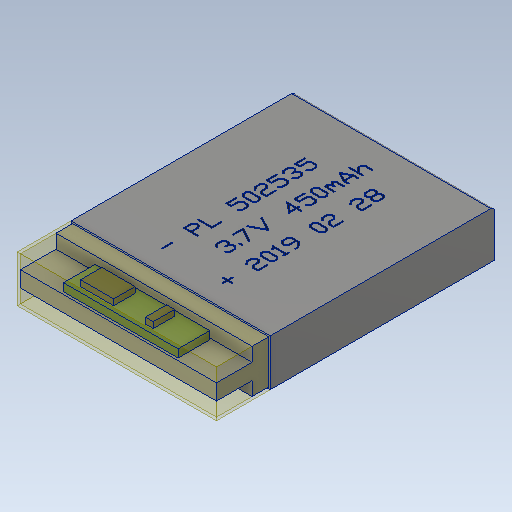
# Autodesk Inventor part: LiPo 502535
Saved by Autodesk Inventor 2020.1 (Build 241239000, 239)
## iProperties
Created: 2019-07-15
Part Number: LiPo 502535
Material: Generic
Document SubType Name: Modeling
Designer: Petar
Density: 1 g/cm^3
Appearance: Default
Mass: 4.91007 g
Surface Area: 36.002 cm^2
Volume: 4.91007 cm^3
Author: Petar
Autodesk Inventor part; units mm, degrees
ref_plane "YZ Plane" through (0, 0, 0) normal (1, 0, 0) x (0, 1, 0)
ref_plane "XZ Plane" through (0, 0, 0) normal (0, 1, 0) x (-1, 0, 0)
sketch "Sketch1" plane through (0, 0, 0) normal (0, 1, 0) x (-1, 0, 0)
  line L0 (-12.6, -17.5205) -> (12.6, -17.5205)
  line L1 (12.6, -17.5205) -> (12.6, 12.9793)
  line L2 (12.5, 17.4793) -> (-12.5, 17.4793)
  line L3 (-12.5, 17.4793) -> (-12.5, 12.9793)
  line L4 (12.5, 12.9793) -> (-12.5, 12.9793)
  line L5 (12.5, 12.9793) -> (12.5, 17.4793)
  line L6 (-12.6, 12.9793) -> (-12.6, -17.5205)
  line L7 (0, -17.5205) -> (0, 12.9793) construction
  line L8 (12.6, 12.9793) -> (12.5, 12.9793)
  line L9 (-12.6, 12.9793) -> (-12.5, 12.9793)
  point P0 (0, 0)
  dimension "d1" = 35
  dimension "d2" = 4.5
  dimension "d12" = 25.2
  dimension "d13" = 25
  constraints: 20 end point, 5 parallel, 4 perpendicular, 2 horizontal, 2 midpoint, 1 collinear, 1 vertical
  measures "d1" distance of L2.start L0.end
  measures "d2" distance between parallel lines of L2 L4
  measures "d12" distance between parallel lines of L6 L1
  measures "d13" distance between parallel lines of L5 L3
extrude "Extrusion1" add sketch "Sketch1" along normal mid plane 5.9 contours L6 L9 L4 L8 L1 L0
extrude "Extrusion2" add sketch "Sketch1" along normal mid plane 2 contours L3 L2 L5 L4
ref_plane "Work Plane1" through (-12.5, 1, 17.6793) normal (0, 0, 1) x (1, 0, 0)
sketch "Sketch3" plane through (-12.5, 1, 17.6793) normal (0, 0, 1) x (1, 0, 0)
  line L0 (25, -2) -> (0, -2) construction
  line L1 (0, -2) -> (0, 0) construction
  line L2 (0, 0) -> (25, 0) construction
  line L3 (25, 0) -> (25, -2) construction
  line L4 (25.1, -3.95) -> (25.1, 1.95) projected
  line L5 (-0.1, 1.95) -> (25.1, 1.95) projected
  line L6 (-0.1, -3.95) -> (-0.1, 1.95) projected
  line L7 (25.1, -3.95) -> (-0.1, -3.95) projected
  line L8 (24.9, 1.75) -> (24.9, -3.75)
  line L9 (24.9, -3.75) -> (0.1, -3.75)
  line L10 (0.1, -3.75) -> (0.1, 1.75)
  line L11 (0.1, 1.75) -> (24.9, 1.75)
  point P0 (12.5, -1)
  dimension "d17" = 0.2
  constraints: 8 end point, 3 other
  measures "d17" distance between parallel lines of L5 L11
extrude "Extrusion4" cut sketch "Sketch3" against normal blind 6.8
extrude "Extrusion5" add sketch "Sketch3" against normal up to next separate body
extrude "Extrusion6" add sketch "Sketch3" against normal blind 0.2 contours L8 L9 L10 L11 bodies 2
sketch "Sketch4" plane through (0, 1, 0) normal (0, 1, 0) x (1, 0, 0)
  line L0 (-7.25, -17.1793) -> (7.25, -17.1793)
  line L1 (7.25, -17.1793) -> (7.25, -13.1793)
  line L2 (7.25, -13.1793) -> (-7.25, -13.1793)
  line L3 (-7.25, -13.1793) -> (-7.25, -17.1793)
  line L4 (0, -17.1793) -> (0, -13.1793) construction
  line L5 (12.4, -17.4793) -> (12.4, -12.9793) construction
  line L6 (-12.4, -12.9793) -> (-12.4, -17.4793) construction
  line L7 (-12.4, -12.9793) -> (12.4, -12.9793) construction
  point P0 (0, 0)
  dimension "d24" = 14.5
  dimension "d25" = 4
  dimension "d26" = 24.8
  dimension "d27" = 12.4
  dimension "d28" = 0.2
  constraints: 10 end point, 2 midpoint, 2 parallel, 1 horizontal, 1 perpendicular
  measures "d24" distance of L2.end L1.end
  measures "d25" distance of L1.end L0.end
  measures "d26" distance between parallel lines of L5 L6
  measures "d27" distance between parallel lines of L5 L4
  measures "d28" distance between parallel lines of L7 L2
extrude "Extrusion7" add sketch "Sketch4" along normal blind 1 bodies 1
sketch "Sketch5" plane through (0, 2, 0) normal (0, 1, 0) x (1, 0, 0)
  line L0 (2.45, -16.5293) -> (3.45, -16.5293)
  line L1 (3.45, -16.5293) -> (3.45, -13.8293)
  line L2 (3.45, -13.8293) -> (2.45, -13.8293)
  line L3 (2.45, -13.8293) -> (2.45, -16.5293)
  line L4 (-5.75, -16.5293) -> (-1.55, -16.5293)
  line L5 (-1.55, -16.5293) -> (-1.55, -13.8293)
  line L6 (-1.55, -13.8293) -> (-5.75, -13.8293)
  line L7 (-5.75, -13.8293) -> (-5.75, -16.5293)
  line L8 (-5.75, -15.1793) -> (-1.55, -15.1793) construction
  line L9 (2.45, -15.1793) -> (3.45, -15.1793) construction
  line L10 (-7.25, -17.1793) -> (7.25, -17.1793) construction
  line L11 (7.25, -17.1793) -> (7.25, -13.1793) construction
  line L12 (-7.25, -13.1793) -> (-7.25, -17.1793) construction
  point P0 (0, 0)
  dimension "d31" = 1
  dimension "d33" = 4.2
  dimension "d34" = 2.7
  dimension "d35" = 2
  dimension "d36" = 3.8
  dimension "d37" = 1.5
  constraints: 20 end point, 5 parallel, 4 midpoint, 2 horizontal, 2 perpendicular, 1 collinear
  measures "d31" distance of L2.end L1.end
  measures "d33" distance of L6.end L5.end
  measures "d34" distance of L5.end L4.end
  measures "d35" distance between parallel lines of L10 L8
  measures "d36" distance between parallel lines of L11 L1
  measures "d37" distance between parallel lines of L12 L7
extrude "Extrusion8" add sketch "Sketch5" along normal up to surface (0.75 mm away) bodies 1
sketch "Sketch6" plane through (0, 2.95, 0) normal (0, 1, 0) x (1, 0, 0)
  line L0 (-12.6, -8.3793) -> (-12.6, 17.5205) construction
  line L1 (-12.6, 17.5205) -> (12.6, 17.5205) construction
  line L2 (12.6, 17.5205) -> (12.6, -8.3793) construction
  line L3 (12.6, -8.3793) -> (-12.6, -8.3793) construction
  line L4 (12.6, 17.5205) -> (-12.6, 17.5205) construction
  line L5 (-12.6, 17.5205) -> (-12.6, -10.8793) construction
  line L6 (12.6, -10.8793) -> (12.6, 17.5205) construction
  line L7 (-12.6, -10.8793) -> (12.6, -10.8793) construction
  line L8 (-3.7334, -6.824) -> (-3.7334, -8.1408)
  line L9 (-3.7334, -8.1408) -> (-3.8859, -8.1408)
  line L10 (-3.8859, -8.1408) -> (-3.8859, -6.824)
  line L11 (-3.8859, -6.824) -> (-3.7334, -6.824)
  line L12 (-4.061, -3.2149) -> (-3.7334, -3.5622)
  line L13 (-3.7334, -3.5622) -> (-3.7334, -4.4109)
  line L14 (-3.7334, -4.4109) -> (-2.9104, -4.4109)
  line L15 (-2.9104, -4.4109) -> (-2.9104, -4.5725)
  line L16 (-2.9104, -4.5725) -> (-4.7285, -4.5725)
  line L17 (-4.7285, -4.5725) -> (-4.7285, -3.5622)
  line L18 (-4.7285, -3.5622) -> (-4.4038, -3.2149)
  line L19 (-4.4038, -3.2149) -> (-4.061, -3.2149)
  line L20 (-4.123, -3.378) -> (-4.3404, -3.378)
  line L21 (-4.3404, -3.378) -> (-4.5775, -3.6287)
  line L22 (-4.5775, -3.6287) -> (-4.5775, -4.4109)
  line L23 (-4.5775, -4.4109) -> (-3.8859, -4.4109)
  line L24 (-3.8859, -4.4109) -> (-3.8859, -3.6287)
  line L25 (-3.8859, -3.6287) -> (-4.123, -3.378)
  line L26 (-2.8938, -1.4421) -> (-2.8938, -2.7785)
  line L27 (-2.8938, -2.7785) -> (-4.7104, -2.7785)
  line L28 (-4.7104, -2.7785) -> (-4.7104, -2.6169)
  line L29 (-4.7104, -2.6169) -> (-3.0433, -2.6169)
  line L30 (-3.0433, -2.6169) -> (-3.0433, -1.4421)
  line L31 (-3.0433, -1.4421) -> (-2.8938, -1.4421)
  line L32 (-3.2169, 2.167) -> (-2.8938, 1.8196)
  line L33 (-2.8938, 1.8196) -> (-2.8938, 1.1552)
  line L34 (-2.8938, 1.1552) -> (-3.235, 0.7883)
  line L35 (-3.235, 0.7883) -> (-3.3438, 0.9045)
  line L36 (-3.3438, 0.9045) -> (-3.0433, 1.2217)
  line L37 (-3.0433, 1.2217) -> (-3.0433, 1.7532)
  line L38 (-3.0433, 1.7532) -> (-3.2788, 2.0039)
  line L39 (-3.2788, 2.0039) -> (-3.7802, 2.0039)
  line L40 (-3.7802, 2.0039) -> (-4.0157, 1.7532)
  line L41 (-4.0157, 1.7532) -> (-4.0157, 0.8094)
  line L42 (-4.0157, 0.8094) -> (-4.7285, 0.8094)
  line L43 (-4.7285, 0.8094) -> (-4.7285, 2.1458)
  line L44 (-4.7285, 2.1458) -> (-4.5775, 2.1458)
  line L45 (-4.5775, 2.1458) -> (-4.5775, 0.971)
  line L46 (-4.5775, 0.971) -> (-4.1683, 0.971)
  line L47 (-4.1683, 0.971) -> (-4.1683, 1.8196)
  line L48 (-4.1683, 1.8196) -> (-3.8421, 2.167)
  line L49 (-3.8421, 2.167) -> (-3.2169, 2.167)
  line L50 (-3.2169, 3.6604) -> (-2.8938, 3.3146)
  line L51 (-2.8938, 3.3146) -> (-2.8938, 2.9492)
  line L52 (-2.8938, 2.9492) -> (-3.2169, 2.6034)
  line L53 (-3.2169, 2.6034) -> (-4.4038, 2.6034)
  line L54 (-4.4038, 2.6034) -> (-4.7285, 2.9492)
  line L55 (-4.7285, 2.9492) -> (-4.7285, 3.3146)
  line L56 (-4.7285, 3.3146) -> (-4.4038, 3.6604)
  line L57 (-4.4038, 3.6604) -> (-3.2169, 3.6604)
  line L58 (-3.2788, 3.4988) -> (-4.3404, 3.4988)
  line L59 (-4.3404, 3.4988) -> (-4.5775, 3.2482)
  line L60 (-4.5775, 3.2482) -> (-4.5775, 3.0156)
  line L61 (-4.5775, 3.0156) -> (-4.3404, 2.765)
  line L62 (-4.3404, 2.765) -> (-3.2788, 2.765)
  line L63 (-3.2788, 2.765) -> (-3.0433, 3.0156)
  line L64 (-3.0433, 3.0156) -> (-3.0433, 3.2482)
  line L65 (-3.0433, 3.2482) -> (-3.2788, 3.4988)
  line L66 (-4.061, 5.4559) -> (-3.7334, 5.1086)
  line L67 (-3.7334, 5.1086) -> (-3.7334, 4.5106)
  line L68 (-3.7334, 4.5106) -> (-3.4978, 4.2599)
  line L69 (-3.4978, 4.2599) -> (-3.0433, 4.2599)
  line L70 (-3.0433, 4.2599) -> (-3.0433, 5.4347)
  line L71 (-3.0433, 5.4347) -> (-2.8938, 5.4347)
  line L72 (-2.8938, 5.4347) -> (-2.8938, 4.0983)
  line L73 (-2.8938, 4.0983) -> (-3.5597, 4.0983)
  line L74 (-3.5597, 4.0983) -> (-3.8859, 4.4441)
  line L75 (-3.8859, 4.4441) -> (-3.8859, 5.0421)
  line L76 (-3.8859, 5.0421) -> (-4.123, 5.2928)
  line L77 (-4.123, 5.2928) -> (-4.3404, 5.2928)
  line L78 (-4.3404, 5.2928) -> (-4.5775, 5.0421)
  line L79 (-4.5775, 5.0421) -> (-4.5775, 4.5106)
  line L80 (-4.5775, 4.5106) -> (-4.277, 4.1935)
  line L81 (-4.277, 4.1935) -> (-4.3857, 4.0772)
  line L82 (-4.3857, 4.0772) -> (-4.7285, 4.4441)
  line L83 (-4.7285, 4.4441) -> (-4.7285, 5.1086)
  line L84 (-4.7285, 5.1086) -> (-4.4038, 5.4559)
  line L85 (-4.4038, 5.4559) -> (-4.061, 5.4559)
  line L86 (-3.2169, 7.2498) -> (-2.8938, 6.9025)
  line L87 (-2.8938, 6.9025) -> (-2.8938, 6.2381)
  line L88 (-2.8938, 6.2381) -> (-3.235, 5.8712)
  line L89 (-3.235, 5.8712) -> (-3.3438, 5.9874)
  line L90 (-3.3438, 5.9874) -> (-3.0433, 6.3045)
  line L91 (-3.0433, 6.3045) -> (-3.0433, 6.8361)
  line L92 (-3.0433, 6.8361) -> (-3.2788, 7.0868)
  line L93 (-3.2788, 7.0868) -> (-3.7802, 7.0868)
  line L94 (-3.7802, 7.0868) -> (-4.0157, 6.8361)
  line L95 (-4.0157, 6.8361) -> (-4.0157, 5.8923)
  line L96 (-4.0157, 5.8923) -> (-4.7285, 5.8923)
  line L97 (-4.7285, 5.8923) -> (-4.7285, 7.2287)
  line L98 (-4.7285, 7.2287) -> (-4.5775, 7.2287)
  line L99 (-4.5775, 7.2287) -> (-4.5775, 6.0539)
  line L100 (-4.5775, 6.0539) -> (-4.1683, 6.0539)
  line L101 (-4.1683, 6.0539) -> (-4.1683, 6.9025)
  line L102 (-4.1683, 6.9025) -> (-3.8421, 7.2498)
  line L103 (-3.8421, 7.2498) -> (-3.2169, 7.2498)
  line L104 (-3.2169, 9.0438) -> (-2.8938, 8.6965)
  line L105 (-2.8938, 8.6965) -> (-2.8938, 8.0321)
  line L106 (-2.8938, 8.0321) -> (-3.235, 7.6651)
  line L107 (-3.235, 7.6651) -> (-3.3438, 7.7814)
  line L108 (-3.3438, 7.7814) -> (-3.0433, 8.0985)
  line L109 (-3.0433, 8.0985) -> (-3.0433, 8.6301)
  line L110 (-3.0433, 8.6301) -> (-3.2788, 8.8807)
  line L111 (-3.2788, 8.8807) -> (-3.4978, 8.8807)
  line L112 (-3.4978, 8.8807) -> (-3.7334, 8.6301)
  line L113 (-3.7334, 8.6301) -> (-3.7334, 8.3039)
  line L114 (-3.7334, 8.3039) -> (-3.8859, 8.3039)
  line L115 (-3.8859, 8.3039) -> (-3.8859, 8.6301)
  line L116 (-3.8859, 8.6301) -> (-4.123, 8.8807)
  line L117 (-4.123, 8.8807) -> (-4.3404, 8.8807)
  line L118 (-4.3404, 8.8807) -> (-4.5775, 8.6301)
  line L119 (-4.5775, 8.6301) -> (-4.5775, 8.0985)
  line L120 (-4.5775, 8.0985) -> (-4.277, 7.7814)
  line L121 (-4.277, 7.7814) -> (-4.3857, 7.6651)
  line L122 (-4.3857, 7.6651) -> (-4.7285, 8.0321)
  line L123 (-4.7285, 8.0321) -> (-4.7285, 8.6965)
  line L124 (-4.7285, 8.6965) -> (-4.4038, 9.0438)
  line L125 (-4.4038, 9.0438) -> (-4.061, 9.0438)
  line L126 (-4.061, 9.0438) -> (-3.8119, 8.7765)
  line L127 (-3.8119, 8.7765) -> (-3.5597, 9.0438)
  line L128 (-3.5597, 9.0438) -> (-3.2169, 9.0438)
  line L129 (-3.2169, 10.8378) -> (-2.8938, 10.4905)
  line L130 (-2.8938, 10.4905) -> (-2.8938, 9.826)
  line L131 (-2.8938, 9.826) -> (-3.235, 9.4591)
  line L132 (-3.235, 9.4591) -> (-3.3438, 9.5754)
  line L133 (-3.3438, 9.5754) -> (-3.0433, 9.8925)
  line L134 (-3.0433, 9.8925) -> (-3.0433, 10.424)
  line L135 (-3.0433, 10.424) -> (-3.2788, 10.6747)
  line L136 (-3.2788, 10.6747) -> (-3.7802, 10.6747)
  line L137 (-3.7802, 10.6747) -> (-4.0157, 10.424)
  line L138 (-4.0157, 10.424) -> (-4.0157, 9.4802)
  line L139 (-4.0157, 9.4802) -> (-4.7285, 9.4802)
  line L140 (-4.7285, 9.4802) -> (-4.7285, 10.8166)
  line L141 (-4.7285, 10.8166) -> (-4.5775, 10.8166)
  line L142 (-4.5775, 10.8166) -> (-4.5775, 9.6418)
  line L143 (-4.5775, 9.6418) -> (-4.1683, 9.6418)
  line L144 (-4.1683, 9.6418) -> (-4.1683, 10.4905)
  line L145 (-4.1683, 10.4905) -> (-3.8421, 10.8378)
  line L146 (-3.8421, 10.8378) -> (-3.2169, 10.8378)
  line L147 (0.5942, -3.2149) -> (0.9174, -3.5622)
  line L148 (0.9174, -3.5622) -> (0.9174, -4.2267)
  line L149 (0.9174, -4.2267) -> (0.5761, -4.5936)
  line L150 (0.5761, -4.5936) -> (0.4674, -4.4773)
  line L151 (0.4674, -4.4773) -> (0.7679, -4.1602)
  line L152 (0.7679, -4.1602) -> (0.7679, -3.6287)
  line L153 (0.7679, -3.6287) -> (0.5323, -3.378)
  line L154 (0.5323, -3.378) -> (0.3133, -3.378)
  line L155 (0.3133, -3.378) -> (0.0778, -3.6287)
  line L156 (0.0778, -3.6287) -> (0.0778, -3.9548)
  line L157 (0.0778, -3.9548) -> (-0.0747, -3.9548)
  line L158 (-0.0747, -3.9548) -> (-0.0747, -3.6287)
  line L159 (-0.0747, -3.6287) -> (-0.3118, -3.378)
  line L160 (-0.3118, -3.378) -> (-0.5293, -3.378)
  line L161 (-0.5293, -3.378) -> (-0.7664, -3.6287)
  line L162 (-0.7664, -3.6287) -> (-0.7664, -4.1602)
  line L163 (-0.7664, -4.1602) -> (-0.4659, -4.4773)
  line L164 (-0.4659, -4.4773) -> (-0.5746, -4.5936)
  line L165 (-0.5746, -4.5936) -> (-0.9174, -4.2267)
  line L166 (-0.9174, -4.2267) -> (-0.9174, -3.5622)
  line L167 (-0.9174, -3.5622) -> (-0.5927, -3.2149)
  line L168 (-0.5927, -3.2149) -> (-0.2499, -3.2149)
  line L169 (-0.2499, -3.2149) -> (-0.0008, -3.4822)
  line L170 (-0.0008, -3.4822) -> (0.2514, -3.2149)
  line L171 (0.2514, -3.2149) -> (0.5942, -3.2149)
  line L172 (0.9008, -2.6169) -> (0.9008, -2.7785)
  line L173 (0.9008, -2.7785) -> (0.5051, -2.7785)
  line L174 (0.5051, -2.7785) -> (0.5051, -2.6169)
  line L175 (0.5051, -2.6169) -> (0.9008, -2.6169)
  line L176 (-0.9174, -0.7731) -> (0.9294, -1.7592)
  line L177 (0.9294, -1.7592) -> (0.8555, -1.8981)
  line L178 (0.8555, -1.8981) -> (-0.7664, -1.0359)
  line L179 (-0.7664, -1.0359) -> (-0.7664, -2.1609)
  line L180 (-0.7664, -2.1609) -> (-0.9174, -2.1609)
  line L181 (-0.9174, -2.1609) -> (-0.9174, -0.7731)
  line L182 (-0.857, 1.5841) -> (0.9008, 0.6493)
  line L183 (0.9008, 0.6493) -> (0.9008, 0.5301)
  line L184 (0.9008, 0.5301) -> (-0.857, -0.4032)
  line L185 (-0.857, -0.4032) -> (-0.9325, -0.2642)
  line L186 (-0.9325, -0.2642) -> (0.6742, 0.5889)
  line L187 (0.6742, 0.5889) -> (-0.931, 1.4421)
  line L188 (-0.931, 1.4421) -> (-0.857, 1.5841)
  line L189 (0.3571, 5.1358) -> (0.3571, 4.8564)
  line L190 (0.3571, 4.8564) -> (0.9008, 4.8564)
  line L191 (0.9008, 4.8564) -> (0.9008, 4.6948)
  line L192 (0.9008, 4.6948) -> (0.3571, 4.6948)
  line L193 (0.3571, 4.6948) -> (0.3571, 3.7178)
  line L194 (0.3571, 3.7178) -> (-1.0699, 4.8564)
  line L195 (-1.0699, 4.8564) -> (0.2046, 4.8564)
  line L196 (0.2046, 4.8564) -> (0.2046, 5.1358)
  line L197 (0.2046, 5.1358) -> (0.3571, 5.1358)
  line L198 (0.2046, 4.6948) -> (-0.6154, 4.6948)
  line L199 (-0.6154, 4.6948) -> (0.2046, 4.041)
  line L200 (0.2046, 4.041) -> (0.2046, 4.6948)
  line L201 (0.5942, 6.9509) -> (0.9174, 6.6035)
  line L202 (0.9174, 6.6035) -> (0.9174, 5.9391)
  line L203 (0.9174, 5.9391) -> (0.5761, 5.5722)
  line L204 (0.5761, 5.5722) -> (0.4674, 5.6884)
  line L205 (0.4674, 5.6884) -> (0.7679, 6.0056)
  line L206 (0.7679, 6.0056) -> (0.7679, 6.5371)
  line L207 (0.7679, 6.5371) -> (0.5323, 6.7878)
  line L208 (0.5323, 6.7878) -> (0.031, 6.7878)
  line L209 (0.031, 6.7878) -> (-0.2046, 6.5371)
  line L210 (-0.2046, 6.5371) -> (-0.2046, 5.5933)
  line L211 (-0.2046, 5.5933) -> (-0.9174, 5.5933)
  line L212 (-0.9174, 5.5933) -> (-0.9174, 6.9297)
  line L213 (-0.9174, 6.9297) -> (-0.7664, 6.9297)
  line L214 (-0.7664, 6.9297) -> (-0.7664, 5.7549)
  line L215 (-0.7664, 5.7549) -> (-0.3571, 5.7549)
  line L216 (-0.3571, 5.7549) -> (-0.3571, 6.6035)
  line L217 (-0.3571, 6.6035) -> (-0.031, 6.9509)
  line L218 (-0.031, 6.9509) -> (0.5942, 6.9509)
  line L219 (0.5942, 8.4443) -> (0.9174, 8.0985)
  line L220 (0.9174, 8.0985) -> (0.9174, 7.7331)
  line L221 (0.9174, 7.7331) -> (0.5942, 7.3873)
  line L222 (0.5942, 7.3873) -> (-0.5927, 7.3873)
  line L223 (-0.5927, 7.3873) -> (-0.9174, 7.7331)
  line L224 (-0.9174, 7.7331) -> (-0.9174, 8.0985)
  line L225 (-0.9174, 8.0985) -> (-0.5927, 8.4443)
  line L226 (-0.5927, 8.4443) -> (0.5942, 8.4443)
  line L227 (0.5323, 8.2827) -> (-0.5293, 8.2827)
  line L228 (-0.5293, 8.2827) -> (-0.7664, 8.0321)
  line L229 (-0.7664, 8.0321) -> (-0.7664, 7.7995)
  line L230 (-0.7664, 7.7995) -> (-0.5293, 7.5488)
  line L231 (-0.5293, 7.5488) -> (0.5323, 7.5488)
  line L232 (0.5323, 7.5488) -> (0.7679, 7.7995)
  line L233 (0.7679, 7.7995) -> (0.7679, 8.0321)
  line L234 (0.7679, 8.0321) -> (0.5323, 8.2827)
  line L235 (0.9008, 10.2398) -> (0.9008, 10.0767)
  line L236 (0.9008, 10.0767) -> (0.031, 10.0767)
  line L237 (0.031, 10.0767) -> (-0.1729, 9.8577)
  line L238 (-0.1729, 9.8577) -> (0.031, 9.6403)
  line L239 (0.031, 9.6403) -> (0.339, 9.6403)
  line L240 (0.339, 9.6403) -> (0.339, 9.4787)
  line L241 (0.339, 9.4787) -> (0.031, 9.4787)
  line L242 (0.031, 9.4787) -> (-0.1729, 9.2613)
  line L243 (-0.1729, 9.2613) -> (0.031, 9.0438)
  line L244 (0.031, 9.0438) -> (0.9008, 9.0438)
  line L245 (0.9008, 9.0438) -> (0.9008, 8.8822)
  line L246 (0.9008, 8.8822) -> (-0.3375, 8.8822)
  line L247 (-0.3375, 8.8822) -> (-0.3375, 9.0438)
  line L248 (-0.3375, 9.0438) -> (-0.1835, 9.0438)
  line L249 (-0.1835, 9.0438) -> (-0.3888, 9.2613)
  line L250 (-0.3888, 9.2613) -> (-0.1065, 9.5603)
  line L251 (-0.1065, 9.5603) -> (-0.3888, 9.8577)
  line L252 (-0.3888, 9.8577) -> (-0.031, 10.2398)
  line L253 (-0.031, 10.2398) -> (0.9008, 10.2398)
  line L254 (0.9008, 12.0337) -> (0.9008, 11.8707)
  line L255 (0.9008, 11.8707) -> (0.3571, 11.8707)
  line L256 (0.3571, 11.8707) -> (0.3571, 10.8378)
  line L257 (0.3571, 10.8378) -> (0.9008, 10.8378)
  line L258 (0.9008, 10.8378) -> (0.9008, 10.6762)
  line L259 (0.9008, 10.6762) -> (0.2635, 10.6762)
  line L260 (0.2635, 10.6762) -> (-0.8992, 11.2938)
  line L261 (-0.8992, 11.2938) -> (-0.8992, 11.4146)
  line L262 (-0.8992, 11.4146) -> (0.2635, 12.0337)
  line L263 (0.2635, 12.0337) -> (0.9008, 12.0337)
  line L264 (0.2046, 11.8208) -> (-0.6712, 11.3542)
  line L265 (-0.6712, 11.3542) -> (0.2046, 10.8876)
  line L266 (0.2046, 10.8876) -> (0.2046, 11.8208)
  line L267 (0.9008, 13.8277) -> (0.9008, 13.6646)
  line L268 (0.9008, 13.6646) -> (0.031, 13.6646)
  line L269 (0.031, 13.6646) -> (-0.2046, 13.4139)
  line L270 (-0.2046, 13.4139) -> (-0.2046, 13.1814)
  line L271 (-0.2046, 13.1814) -> (0.3133, 12.6317)
  line L272 (0.3133, 12.6317) -> (0.9008, 12.6317)
  line L273 (0.9008, 12.6317) -> (0.9008, 12.4702)
  line L274 (0.9008, 12.4702) -> (-0.8992, 12.4702)
  line L275 (-0.8992, 12.4702) -> (-0.8992, 12.6317)
  line L276 (-0.8992, 12.6317) -> (0.0974, 12.6317)
  line L277 (0.0974, 12.6317) -> (-0.3571, 13.115)
  line L278 (-0.3571, 13.115) -> (-0.3571, 13.4804)
  line L279 (-0.3571, 13.4804) -> (-0.031, 13.8277)
  line L280 (-0.031, 13.8277) -> (0.9008, 13.8277)
  line L281 (3.8889, -6.824) -> (3.8889, -7.4023)
  line L282 (3.8889, -7.4023) -> (4.431, -7.4023)
  line L283 (4.431, -7.4023) -> (4.431, -7.5639)
  line L284 (4.431, -7.5639) -> (3.8889, -7.5639)
  line L285 (3.8889, -7.5639) -> (3.8889, -8.1408)
  line L286 (3.8889, -8.1408) -> (3.7364, -8.1408)
  line L287 (3.7364, -8.1408) -> (3.7364, -7.5639)
  line L288 (3.7364, -7.5639) -> (3.1928, -7.5639)
  line L289 (3.1928, -7.5639) -> (3.1928, -7.4023)
  line L290 (3.1928, -7.4023) -> (3.7364, -7.4023)
  line L291 (3.7364, -7.4023) -> (3.7364, -6.824)
  line L292 (3.7364, -6.824) -> (3.8889, -6.824)
  line L293 (3.5612, -3.2149) -> (3.8889, -3.5622)
  line L294 (3.8889, -3.5622) -> (3.8889, -4.1602)
  line L295 (3.8889, -4.1602) -> (4.1245, -4.4109)
  line L296 (4.1245, -4.4109) -> (4.579, -4.4109)
  line L297 (4.579, -4.4109) -> (4.579, -3.2361)
  line L298 (4.579, -3.2361) -> (4.7285, -3.2361)
  line L299 (4.7285, -3.2361) -> (4.7285, -4.5725)
  line L300 (4.7285, -4.5725) -> (4.0626, -4.5725)
  line L301 (4.0626, -4.5725) -> (3.7364, -4.2267)
  line L302 (3.7364, -4.2267) -> (3.7364, -3.6287)
  line L303 (3.7364, -3.6287) -> (3.4993, -3.378)
  line L304 (3.4993, -3.378) -> (3.2819, -3.378)
  line L305 (3.2819, -3.378) -> (3.0448, -3.6287)
  line L306 (3.0448, -3.6287) -> (3.0448, -4.1602)
  line L307 (3.0448, -4.1602) -> (3.3453, -4.4773)
  line L308 (3.3453, -4.4773) -> (3.2366, -4.5936)
  line L309 (3.2366, -4.5936) -> (2.8938, -4.2267)
  line L310 (2.8938, -4.2267) -> (2.8938, -3.5622)
  line L311 (2.8938, -3.5622) -> (3.2184, -3.2149)
  line L312 (3.2184, -3.2149) -> (3.5612, -3.2149)
  line L313 (4.4053, -1.7215) -> (4.7285, -2.0673)
  line L314 (4.7285, -2.0673) -> (4.7285, -2.4327)
  line L315 (4.7285, -2.4327) -> (4.4053, -2.7785)
  line L316 (4.4053, -2.7785) -> (3.2184, -2.7785)
  line L317 (3.2184, -2.7785) -> (2.8938, -2.4327)
  line L318 (2.8938, -2.4327) -> (2.8938, -2.0673)
  line L319 (2.8938, -2.0673) -> (3.2184, -1.7215)
  line L320 (3.2184, -1.7215) -> (4.4053, -1.7215)
  line L321 (4.3434, -1.883) -> (3.2819, -1.883)
  line L322 (3.2819, -1.883) -> (3.0448, -2.1337)
  line L323 (3.0448, -2.1337) -> (3.0448, -2.3663)
  line L324 (3.0448, -2.3663) -> (3.2819, -2.6169)
  line L325 (3.2819, -2.6169) -> (4.3434, -2.6169)
  line L326 (4.3434, -2.6169) -> (4.579, -2.3663)
  line L327 (4.579, -2.3663) -> (4.579, -2.1337)
  line L328 (4.579, -2.1337) -> (4.3434, -1.883)
  line L329 (4.7285, -0.5451) -> (4.7285, -1.2639)
  line L330 (4.7285, -1.2639) -> (4.579, -1.2639)
  line L331 (4.579, -1.2639) -> (4.579, -0.9845)
  line L332 (4.579, -0.9845) -> (3.152, -0.9845)
  line L333 (3.152, -0.9845) -> (3.3453, -1.1884)
  line L334 (3.3453, -1.1884) -> (3.2366, -1.3047)
  line L335 (3.2366, -1.3047) -> (2.8938, -0.9377)
  line L336 (2.8938, -0.9377) -> (2.8938, -0.8245)
  line L337 (2.8938, -0.8245) -> (4.579, -0.8245)
  line L338 (4.579, -0.8245) -> (4.579, -0.5451)
  line L339 (4.579, -0.5451) -> (4.7285, -0.5451)
  line L340 (4.1245, 1.27) -> (4.7285, 0.6237)
  line L341 (4.7285, 0.6237) -> (4.7285, 0.2311)
  line L342 (4.7285, 0.2311) -> (4.579, 0.2311)
  line L343 (4.579, 0.2311) -> (4.579, 0.5572)
  line L344 (4.579, 0.5572) -> (4.0626, 1.1069)
  line L345 (4.0626, 1.1069) -> (3.8889, 1.1069)
  line L346 (3.8889, 1.1069) -> (3.8889, 0.2582)
  line L347 (3.8889, 0.2582) -> (3.5612, -0.0876)
  line L348 (3.5612, -0.0876) -> (3.2184, -0.0876)
  line L349 (3.2184, -0.0876) -> (2.8938, 0.2582)
  line L350 (2.8938, 0.2582) -> (2.8938, 0.9227)
  line L351 (2.8938, 0.9227) -> (3.2184, 1.27)
  line L352 (3.2184, 1.27) -> (4.1245, 1.27)
  line L353 (3.7364, 1.1069) -> (3.2819, 1.1069)
  line L354 (3.2819, 1.1069) -> (3.0448, 0.8562)
  line L355 (3.0448, 0.8562) -> (3.0448, 0.3247)
  line L356 (3.0448, 0.3247) -> (3.2819, 0.074)
  line L357 (3.2819, 0.074) -> (3.4993, 0.074)
  line L358 (3.4993, 0.074) -> (3.7364, 0.3247)
  line L359 (3.7364, 0.3247) -> (3.7364, 1.1069)
  line L360 (4.4053, 4.5574) -> (4.7285, 4.2116)
  line L361 (4.7285, 4.2116) -> (4.7285, 3.8462)
  line L362 (4.7285, 3.8462) -> (4.4053, 3.5004)
  line L363 (4.4053, 3.5004) -> (3.2184, 3.5004)
  line L364 (3.2184, 3.5004) -> (2.8938, 3.8462)
  line L365 (2.8938, 3.8462) -> (2.8938, 4.2116)
  line L366 (2.8938, 4.2116) -> (3.2184, 4.5574)
  line L367 (3.2184, 4.5574) -> (4.4053, 4.5574)
  line L368 (4.3434, 4.3958) -> (3.2819, 4.3958)
  line L369 (3.2819, 4.3958) -> (3.0448, 4.1452)
  line L370 (3.0448, 4.1452) -> (3.0448, 3.9126)
  line L371 (3.0448, 3.9126) -> (3.2819, 3.6619)
  line L372 (3.2819, 3.6619) -> (4.3434, 3.6619)
  line L373 (4.3434, 3.6619) -> (4.579, 3.9126)
  line L374 (4.579, 3.9126) -> (4.579, 4.1452)
  line L375 (4.579, 4.1452) -> (4.3434, 4.3958)
  line L376 (3.5612, 6.3529) -> (3.8889, 6.0056)
  line L377 (3.8889, 6.0056) -> (3.8889, 5.4076)
  line L378 (3.8889, 5.4076) -> (4.1245, 5.1569)
  line L379 (4.1245, 5.1569) -> (4.579, 5.1569)
  line L380 (4.579, 5.1569) -> (4.579, 6.3317)
  line L381 (4.579, 6.3317) -> (4.7285, 6.3317)
  line L382 (4.7285, 6.3317) -> (4.7285, 4.9953)
  line L383 (4.7285, 4.9953) -> (4.0626, 4.9953)
  line L384 (4.0626, 4.9953) -> (3.7364, 5.3411)
  line L385 (3.7364, 5.3411) -> (3.7364, 5.9391)
  line L386 (3.7364, 5.9391) -> (3.4993, 6.1898)
  line L387 (3.4993, 6.1898) -> (3.2819, 6.1898)
  line L388 (3.2819, 6.1898) -> (3.0448, 5.9391)
  line L389 (3.0448, 5.9391) -> (3.0448, 5.4076)
  line L390 (3.0448, 5.4076) -> (3.3453, 5.0905)
  line L391 (3.3453, 5.0905) -> (3.2366, 4.9742)
  line L392 (3.2366, 4.9742) -> (2.8938, 5.3411)
  line L393 (2.8938, 5.3411) -> (2.8938, 6.0056)
  line L394 (2.8938, 6.0056) -> (3.2184, 6.3529)
  line L395 (3.2184, 6.3529) -> (3.5612, 6.3529)
  line L396 (3.5612, 9.9408) -> (3.8889, 9.5935)
  line L397 (3.8889, 9.5935) -> (3.8889, 8.9955)
  line L398 (3.8889, 8.9955) -> (4.1245, 8.7448)
  line L399 (4.1245, 8.7448) -> (4.579, 8.7448)
  line L400 (4.579, 8.7448) -> (4.579, 9.9196)
  line L401 (4.579, 9.9196) -> (4.7285, 9.9196)
  line L402 (4.7285, 9.9196) -> (4.7285, 8.5832)
  line L403 (4.7285, 8.5832) -> (4.0626, 8.5832)
  line L404 (4.0626, 8.5832) -> (3.7364, 8.929)
  line L405 (3.7364, 8.929) -> (3.7364, 9.527)
  line L406 (3.7364, 9.527) -> (3.4993, 9.7777)
  line L407 (3.4993, 9.7777) -> (3.2819, 9.7777)
  line L408 (3.2819, 9.7777) -> (3.0448, 9.527)
  line L409 (3.0448, 9.527) -> (3.0448, 8.9955)
  line L410 (3.0448, 8.9955) -> (3.3453, 8.6784)
  line L411 (3.3453, 8.6784) -> (3.2366, 8.5621)
  line L412 (3.2366, 8.5621) -> (2.8938, 8.929)
  line L413 (2.8938, 8.929) -> (2.8938, 9.5935)
  line L414 (2.8938, 9.5935) -> (3.2184, 9.9408)
  line L415 (3.2184, 9.9408) -> (3.5612, 9.9408)
  line L416 (4.4053, 11.7347) -> (4.7285, 11.3874)
  line L417 (4.7285, 11.3874) -> (4.7285, 10.723)
  line L418 (4.7285, 10.723) -> (4.4053, 10.3772)
  line L419 (4.4053, 10.3772) -> (4.0626, 10.3772)
  line L420 (4.0626, 10.3772) -> (3.8104, 10.6415)
  line L421 (3.8104, 10.6415) -> (3.5612, 10.3772)
  line L422 (3.5612, 10.3772) -> (3.2184, 10.3772)
  line L423 (3.2184, 10.3772) -> (2.8938, 10.723)
  line L424 (2.8938, 10.723) -> (2.8938, 11.3874)
  line L425 (2.8938, 11.3874) -> (3.2184, 11.7347)
  line L426 (3.2184, 11.7347) -> (3.5612, 11.7347)
  line L427 (3.5612, 11.7347) -> (3.8104, 11.4675)
  line L428 (3.8104, 11.4675) -> (4.0626, 11.7347)
  line L429 (4.0626, 11.7347) -> (4.4053, 11.7347)
  line L430 (3.4993, 11.5717) -> (3.2819, 11.5717)
  line L431 (3.2819, 11.5717) -> (3.0448, 11.321)
  line L432 (3.0448, 11.321) -> (3.0448, 10.7894)
  line L433 (3.0448, 10.7894) -> (3.2819, 10.5388)
  line L434 (3.2819, 10.5388) -> (3.4993, 10.5388)
  line L435 (3.4993, 10.5388) -> (3.7364, 10.7894)
  line L436 (3.7364, 10.7894) -> (3.7364, 11.321)
  line L437 (3.7364, 11.321) -> (3.4993, 11.5717)
  line L438 (4.3434, 11.5717) -> (4.1245, 11.5717)
  line L439 (4.1245, 11.5717) -> (3.8889, 11.321)
  line L440 (3.8889, 11.321) -> (3.8889, 10.7894)
  line L441 (3.8889, 10.7894) -> (4.1245, 10.5388)
  line L442 (4.1245, 10.5388) -> (4.3434, 10.5388)
  line L443 (4.3434, 10.5388) -> (4.579, 10.7894)
  line L444 (4.579, 10.7894) -> (4.579, 11.321)
  line L445 (4.579, 11.321) -> (4.3434, 11.5717)
  point P0 (0, 0)
  dimension "d40" = 2.5
  constraints: 3 collinear, 2 other
  measures "d40" distance between parallel lines of L7 L3
emboss "Emboss1" sketch "Sketch6" operation cut depth 0.001 direction (0, -1, 0)
fillet "Fillet3" radius 0.5 1 edges at (0, 2.95, -17.5205)
equation "\"d27\" = 0.5 * d26"
body "Solid1"
body "Solid3"
